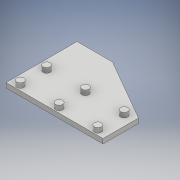
# Autodesk Inventor part: Wheels
Saved by Autodesk Inventor 2017 (Build 210142000, 142)
## iProperties
Created: 2016-12-07
Part Number: Wheels
Material: Generic
Document SubType Name: Modeling
Designer: umr
Density: 1 g/cm^3
Appearance: Default
Author: umr
Autodesk Inventor part; units mm, degrees
ref_plane "YZ Plane" through (0, 0, 0) normal (1, 0, 0) x (0, 1, 0)
ref_plane "XZ Plane" through (0, 0, 0) normal (0, 1, 0) x (-1, 0, 0)
ref_plane "XY Plane" through (0, 0, 0) normal (0, 0, 1) x (1, 0, 0)
sketch "Sketch1" plane through (0, 0, 0) normal (0, 0, 1) x (1, 0, 0)
  line L0 (0, 0) -> (204.9038, 0)
  line L1 (75, 150) -> (0, 150)
  line L2 (0, 150) -> (0, 0)
  line L3 (204.9038, 0) -> (204.9038, 75)
  line L4 (75, 150) -> (204.9038, 75)
  dimension "d0" = 150
  dimension "d2" = 75
  dimension "d6" = 90
  dimension "d9" = 150
  dimension "d10" = 90
  dimension "d11" = 75
  constraints: 10 end point, 1 horizontal, 1 parallel
  measures "d0" distance of L1.end L0.start
  measures "d2" distance of L1.start L1.end
  measures "d6" angle of L0 L2
  measures "d9" angle of L4 L1
  measures "d10" angle of L0 L3
  measures "d11" distance of L0.end L3.end
extrude "Extrusion1" add sketch "Sketch1" along normal blind 10
sketch "Sketch2" plane through (0, 0, 10) normal (0, 0, 1) x (1, 0, 0)
  line L0 (204.9038, 0) -> (204.9038, 75) projected
  line L1 (204.9038, 37.5) -> (0, 37.5)
  line L2 (0, 150) -> (0, 0) projected
  circle A0 centre (20.4904, 65.2778) radius 7.5
  circle A1 centre (102.4519, 65.2778) radius 7.5
  circle A2 centre (184.4134, 65.2778) radius 7.5
  circle A3 centre (20.4904, 9.7222) radius 7.5
  circle A4 centre (102.4519, 9.7222) radius 7.5
  circle A5 centre (184.4134, 9.7222) radius 7.5
  dimension "d12" = 15
  dimension "d13" = 75
  dimension "d15" = 204.9038
  dimension "d16" = 20.4904
  dimension "d17" = 27.7778
  dimension "d20" = 81.9615
  dimension "d23" = 55.5556
  constraints: 6 centre point, 2 end point, 2 horizontal, 1 midpoint, 1 point on line, 1 vertical, 10 other
  measures "d12" diameter of A0
  measures "d13" distance of L0.start L0.end
  measures "d15" distance of L1.start L1.end
  measures "d16" distance from line of L2 A0.centre
  measures "d17" distance from line of L1 A0.centre
  measures "d20" distance of A0.centre A1.centre
  measures "d23" distance of A0.centre A3.centre
extrude "Extrusion2" add sketch "Sketch2" along normal blind 10
equation "\"d2\" = 0.5 * d0"
equation "\"d11\" = 0.5 * d0"
equation "\"d12\" = 0.2 * d13"
equation "\"d16\" = 0.1 * d15"
equation "\"d17\" = 0.37037 * d13"
equation "\"d20\" = -d16 + 0.5 * d15"
equation "\"d23\" = 2 * d17"
body "Solid1"
